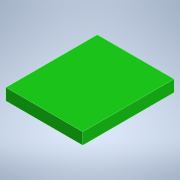
# Autodesk Inventor part: StartModuleBoard
Saved by Autodesk Inventor 2021 (Build 250183000, 183)
## iProperties
Created: 2021-09-12
Part Number: StartModuleBoard
Material: Generic
Document SubType Name: Modeling
Designer: ermoz
Density: 1 g/cm^3
Appearance: Default
Author: ermoz
Autodesk Inventor part; units mm, degrees
ref_plane "YZ Plane" through (0, 0, 0) normal (1, 0, 0) x (0, 1, 0)
ref_plane "XZ Plane" through (0, 0, 0) normal (0, 1, 0) x (-1, 0, 0)
ref_plane "XY Plane" through (0, 0, 0) normal (0, 0, 1) x (1, 0, 0)
sketch "Sketch1" plane through (0, 0, 0) normal (0, 1, 0) x (-1, 0, 0)
  line L0 (-5.25, -6.25) -> (5.25, -6.25)
  line L1 (5.25, -6.25) -> (5.25, 6.25)
  line L2 (5.25, 6.25) -> (-5.25, 6.25)
  line L3 (-5.25, 6.25) -> (-5.25, -6.25)
  line L4 (-5.25, -6.25) -> (5.25, 6.25) construction
  line L5 (5.25, -6.25) -> (-5.25, 6.25) construction
  point P0 (0, 0)
  dimension "d0" = 10.5
  dimension "d1" = 12.5
  constraints: 12 end point, 2 midpoint, 2 parallel, 1 horizontal, 1 perpendicular
  measures "d0" distance of L2.end L1.end
  measures "d1" distance of L1.end L0.end
extrude "Extrusion1" add sketch "Sketch1" along normal blind 1.6
body "Solid1"
